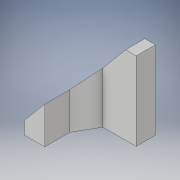
# Autodesk Inventor part: 複習二
Saved by Autodesk Inventor 2017 (Build 210142000, 142)
## iProperties
Part Number: 複習二
Material: 一般
Document SubType Name: Modeling
Designer: user
Density: 1 g/cm^3
Appearance: 預設
Author: user
Autodesk Inventor part; units mm, degrees
ref_plane "YZ Plane" through (0, 0, 0) normal (1, 0, 0) x (0, 1, 0)
ref_plane "XZ Plane" through (0, 0, 0) normal (0, 1, 0) x (-1, 0, 0)
ref_plane "XY Plane" through (0, 0, 0) normal (0, 0, 1) x (1, 0, 0)
sketch "草圖1" plane through (0, 0, 0) normal (0, 1, 0) x (-1, 0, 0)
  line L0 (0, 0) -> (-23, 0)
  line L1 (-23, 0) -> (-23, -29)
  line L2 (-23, -29) -> (-36.8564, -53)
  line L3 (-36.8564, -53) -> (-75, -53)
  line L4 (-75, -53) -> (-75, -75)
  line L5 (-75, -75) -> (-23, -75)
  line L6 (-23, -75) -> (0, -35.1628)
  line L7 (0, -35.1628) -> (0, 0)
  dimension "d1" = 23
  dimension "d2" = 75
  dimension "d3" = 23
  dimension "d4" = 22
  dimension "d5" = 120
  dimension "d6" = 75
  constraints: 16 end point, 3 parallel, 3 perpendicular, 1 horizontal, 1 point on line
  measures "d1" distance of L0.start L0.end
  measures "d2" distance between parallel lines of L4 L7
  measures "d3" distance between parallel lines of L2 L6
  measures "d4" distance of L3.end L4.end
  measures "d5" angle of L3 L2
  measures "d6" distance between parallel lines of L5 L0
extrude "擠出1" add sketch "草圖1" along normal blind 90
sketch "草圖2" plane through (0, 0, 0) normal (0, 0, 1) x (1, 0, 0)
  line L0 (0, 15) -> (63, 90)
  line L1 (36.8564, 90) -> (75, 90) projected
  line L2 (23, 90) -> (0, 90) projected
  line L3 (63, 90) -> (0, 90)
  line L4 (0, 90) -> (0, 15)
  line L5 (75, 0) -> (75, 90) projected
  point P0 (0, 0)
  dimension "d9" = 12
  dimension "d10" = 15
  constraints: 6 end point, 1 horizontal, 1 perpendicular, 1 point on line
  measures "d9" distance from line of L5 L0.end
  measures "d10" distance of point (0, 0) L0.start
extrude "擠出2" cut sketch "草圖2" against normal up to next
